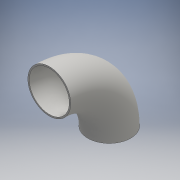
# Autodesk Inventor part: joelho 90 10 inch ANSI B16.9
Saved by Autodesk Inventor 2016 (Build 200138000, 138)
## iProperties
Created: 2018-09-12
Part Number: joelho 90 10 inch ANSI B16.9
Material: Generic
Document SubType Name: Modeling
Designer: User
Density: 1 g/cm^3
Appearance: Default
Author: User
Autodesk Inventor part; units mm, degrees
ref_plane "YZ Plane" through (0, 0, 0) normal (1, 0, 0) x (0, 1, 0)
ref_plane "XZ Plane" through (0, 0, 0) normal (0, 1, 0) x (-1, 0, 0)
ref_plane "XY Plane" through (0, 0, 0) normal (0, 0, 1) x (1, 0, 0)
sketch "Sketch3" plane through (0, 0, 0) normal (0, 1, 0) x (-1, 0, 0)
  circle A0 centre (0, 381) radius 136.5
  circle A1 centre (0, 381) radius 127.23
  point P0 (0, 228.5)
  point P1 (0, 0)
  dimension "d14" = 273
  dimension "d15" = 9.27
  constraints: 2 centre point, 1 coincident
  measures "d14" diameter of A0
  measures "d15" radial gap between concentric circles of A0 A1
sketch "Sketch2" plane through (0, 0, 0) normal (1, 0, 0) x (0, 1, 0)
  arc A0 (381, 0) -> (0, 381) centre (0, 0) ccw
  constraints: 2 point on circle, 1 centre point, 1 coincident
sweep "Sweep2" add profiles "Sketch3" path "Sketch2"
body "Solid2"
